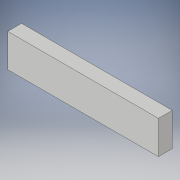
# Autodesk Inventor part: Chain link
Saved by Autodesk Inventor 2019 (Build 230136000, 136)
## iProperties
Created: 2018-12-10
Part Number: Chain link
Material: Generic
Document SubType Name: Modeling
Designer: scigu
Density: 1 g/cm^3
Appearance: Default
Mass: 1.11774 g
Surface Area: 9.64082 cm^2
Volume: 1.11774 cm^3
Author: scigu
Autodesk Inventor part; units mm, degrees
ref_plane "YZ Plane" through (0, 0, 0) normal (1, 0, 0) x (0, 1, 0)
ref_plane "XZ Plane" through (0, 0, 0) normal (0, 1, 0) x (-1, 0, 0)
ref_plane "XY Plane" through (0, 0, 0) normal (0, 0, 1) x (1, 0, 0)
sketch "Sketch1" plane through (0, 0, 0) normal (1, 0, 0) x (0, 1, 0)
  line L0 (-4.191, -1.75) -> (4.191, -1.75)
  line L1 (4.191, -1.75) -> (4.191, 1.75)
  line L2 (4.191, 1.75) -> (-4.191, 1.75)
  line L3 (-4.191, 1.75) -> (-4.191, -1.75)
  line L4 (-4.191, -1.75) -> (4.191, 1.75) construction
  line L5 (4.191, -1.75) -> (-4.191, 1.75) construction
  point P0 (0, 0)
  dimension "d0" = 8.382
  dimension "d1" = 3.5
  constraints: 12 end point, 2 midpoint, 2 parallel, 1 horizontal, 1 perpendicular
  measures "d0" distance of L2.end L1.end
  measures "d1" distance of L1.end L0.end
extrude "Extrusion1" add sketch "Sketch1" along normal mid plane 38.1
body "Solid1"
